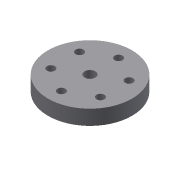
# Autodesk Inventor part: Window Motor Adapter
Saved by Autodesk Inventor 2015 (Build 190159000, 159)
## iProperties
Created: 2016-03-31
Part Number: Window Motor Adapter
Material: Generic
Document SubType Name: Modeling
Designer: Peter
Density: 1 g/cm^3
Appearance: Default
Author: Peter
Autodesk Inventor part; units mm, degrees
ref_plane "YZ Plane" through (0, 0, 0) normal (1, 0, 0) x (0, 1, 0)
sketch "Sketch1" plane through (0, 0, 0) normal (0, 0, 1) x (1, 0, 0)
  circle A0 centre (0, 0) radius 18.33
  arc A1 (-1.8, 7.7127) -> (-3.5788, 7.0653) centre (0, 0) ccw
  arc A2 (3.5788, 7.0653) -> (1.8, 7.7127) centre (0, 0) ccw
  arc A3 (7.3109, 3.0458) -> (6.3365, 4.7513) centre (0, 0) ccw
  arc A4 (7.5794, -2.2975) -> (7.9081, -0.4334) centre (0, 0) ccw
  arc A5 (4.3294, -6.632) -> (5.7794, -5.4152) centre (0, 0) ccw
  arc A6 (-0.9465, -7.8632) -> (0.9465, -7.8632) centre (0, 0) ccw
  arc A7 (-5.7794, -5.4152) -> (-4.3294, -6.632) centre (0, 0) ccw
  arc A8 (-6.3365, 4.7513) -> (-7.283, 3.112) centre (0, 0) ccw
  arc A9 (-7.9081, -0.4334) -> (-7.5794, -2.2975) centre (0, 0) ccw
  line L0 (-0.9465, -7.8632) -> (-2.2366, -11.4078)
  line L1 (-4.3294, -6.632) -> (-5.6195, -10.1765)
  line L2 (-5.6195, -10.1765) -> (-4.5495, -12.0298)
  line L3 (-2.2366, -11.4078) -> (-4.2475, -12.1397)
  arc A10 (-4.5495, -12.0298) -> (-4.2475, -12.1397) centre (-4.333, -11.9048) ccw
  line L4 (4.3294, -6.632) -> (5.6195, -10.1765)
  line L5 (0.9465, -7.8632) -> (2.2366, -11.4078)
  line L6 (2.2366, -11.4078) -> (4.2475, -12.1397)
  line L7 (5.6195, -10.1765) -> (4.5495, -12.0298)
  arc A11 (4.2475, -12.1397) -> (4.5495, -12.0298) centre (4.333, -11.9048) ccw
  line L8 (7.5794, -2.2975) -> (10.8461, -4.1836)
  line L9 (5.7794, -5.4152) -> (9.0461, -7.3012)
  line L10 (9.0461, -7.3012) -> (11.057, -6.5693)
  line L11 (10.8461, -4.1836) -> (11.2177, -6.291)
  arc A12 (11.057, -6.5693) -> (11.2177, -6.291) centre (10.9715, -6.3344) ccw
  line L12 (7.283, 3.112) -> (10.9978, 3.767)
  line L13 (7.9081, -0.4334) -> (11.6229, 0.2217)
  line L14 (11.6229, 0.2217) -> (12.6929, 2.0749)
  line L15 (10.9978, 3.767) -> (12.6371, 2.3914)
  arc A13 (12.6929, 2.0749) -> (12.6371, 2.3914) centre (12.4764, 2.1999) ccw
  line L16 (3.5788, 7.0653) -> (6.0034, 9.9549)
  line L17 (6.3365, 4.7513) -> (8.7612, 7.6408)
  line L18 (8.7612, 7.6408) -> (8.3896, 9.7483)
  line L19 (6.0034, 9.9549) -> (8.1434, 9.9549)
  arc A14 (8.3896, 9.7483) -> (8.1434, 9.9549) centre (8.1434, 9.7049) ccw
  line L20 (-1.8, 7.7127) -> (-1.8, 11.4848)
  line L21 (1.8, 7.7127) -> (1.8, 11.4848)
  line L22 (1.8, 11.4848) -> (0.1607, 12.8603)
  line L23 (-1.8, 11.4848) -> (-0.1607, 12.8603)
  arc A15 (0.1607, 12.8603) -> (-0.1607, 12.8603) centre (0, 12.6688) ccw
  line L24 (-6.3365, 4.7513) -> (-8.7612, 7.6408)
  line L25 (-3.5788, 7.0653) -> (-6.0034, 9.9549)
  line L26 (-6.0034, 9.9549) -> (-8.1434, 9.9549)
  line L27 (-8.7612, 7.6408) -> (-8.3896, 9.7483)
  arc A16 (-8.1434, 9.9549) -> (-8.3896, 9.7483) centre (-8.1434, 9.7049) ccw
  line L28 (-7.9081, -0.4334) -> (-11.6229, 0.2217)
  line L29 (-7.283, 3.112) -> (-10.9978, 3.767)
  line L30 (-10.9978, 3.767) -> (-12.6371, 2.3914)
  line L31 (-11.6229, 0.2217) -> (-12.6929, 2.0749)
  arc A17 (-12.6371, 2.3914) -> (-12.6929, 2.0749) centre (-12.4764, 2.1999) ccw
  line L32 (-5.7794, -5.4152) -> (-9.0461, -7.3012)
  line L33 (-7.5794, -2.2975) -> (-10.8461, -4.1836)
  line L34 (-10.8461, -4.1836) -> (-11.2177, -6.291)
  line L35 (-9.0461, -7.3012) -> (-11.057, -6.5693)
  arc A18 (-11.2177, -6.291) -> (-11.057, -6.5693) centre (-10.9715, -6.3344) ccw
  arc A19 (-0.9465, -7.8632) -> (0.9465, -7.8632) centre (0, 0) ccw
  arc A20 (4.3294, -6.632) -> (5.7794, -5.4152) centre (0, 0) ccw
  arc A21 (7.5794, -2.2975) -> (7.9081, -0.4334) centre (0, 0) ccw
  arc A22 (7.283, 3.112) -> (6.3365, 4.7513) centre (0, 0) ccw
  arc A23 (3.5788, 7.0653) -> (1.8, 7.7127) centre (0, 0) ccw
  arc A24 (-1.8, 7.7127) -> (-3.5788, 7.0653) centre (0, 0) ccw
  arc A25 (-6.3365, 4.7513) -> (-7.283, 3.112) centre (0, 0) ccw
  arc A26 (-7.9081, -0.4334) -> (-7.5794, -2.2975) centre (0, 0) ccw
  arc A27 (-5.7794, -5.4152) -> (-4.3294, -6.632) centre (0, 0) ccw
  point P0 (-2.306, -11.394)
  point P1 (-5.5574, -10.2106)
  dimension "d58" = 0.25
  dimension "d61" = 360
  constraints: 72 end point, 54 point on circle, 28 centre point, 2 coincident, 2 tangent, 109 other
  measures "d58" radius of A10
ref_plane "Work Plane1" through (0, 0, 10) normal (0, 0, 1) x (1, 0, 0)
sketch "Sketch2" plane through (0, 0, 10) normal (0, 0, 1) x (1, 0, 0)
  circle A0 centre (0, 0) radius 34.925
  circle A1 centre (0, 23.8125) radius 3.302
  circle A2 centre (-20.6222, 11.9063) radius 3.302
  circle A3 centre (-20.6222, -11.9062) radius 3.302
  circle A4 centre (0, -23.8125) radius 3.302
  circle A5 centre (20.6222, -11.9063) radius 3.302
  circle A6 centre (20.6222, 11.9062) radius 3.302
  dimension "d42" = 69.85
  dimension "d44" = 6.604
  dimension "d47" = 360
  constraints: 7 centre point, 1 coincident, 13 other
  measures "d42" diameter of A0
  measures "d44" diameter of A1
extrude "Extrusion2" add sketch "Sketch2" along normal blind 6.35
ref_plane "Work Plane2" through (0, 0, 10) normal (0, 0, -1) x (-1, 0, 0)
extrude "Extrusion4" add sketch "Sketch1" along normal up to surface (10 mm away)
sketch "Sketch4" plane through (0, 0, 10) normal (0, 0, -1) x (-1, 0, 0)
  circle A0 centre (0, 0) radius 4.5
  dimension "d65" = 9
  constraints: 1 centre point, 1 coincident
  measures "d65" diameter of A0
extrude "Extrusion5" cut sketch "Sketch4" against normal blind 10
fillet "Fillet1" radius 2 1 edges at (-18.33, 0, 10)
sketch "Sketch6" plane through (0, 0, 16.35) normal (0, 0, 1) x (1, 0, 0)
  circle A0 centre (0, 0) radius 34.925
  circle A1 centre (0, -23.8125) radius 3.302 projected
  circle A2 centre (0, -23.8125) radius 3.302
  circle A3 centre (20.6222, -11.9063) radius 3.302
  circle A4 centre (20.6222, 11.9062) radius 3.302
  circle A5 centre (0, 23.8125) radius 3.302
  circle A6 centre (-20.6222, 11.9063) radius 3.302
  circle A7 centre (-20.6222, -11.9062) radius 3.302
  dimension "d77" = 360
  constraints: 7 centre point, 2 coincident, 13 other
extrude "Extrusion7" add sketch "Sketch6" along normal blind 6.05
sketch "Sketch7" plane through (0, 0, 16.35) normal (0, 0, -1) x (-1, 0, 0)
  circle A0 centre (0, 0) radius 4.5
  constraints: 1 centre point, 1 coincident
extrude "Extrusion8" cut sketch "Sketch7" against normal up to surface (6.05 mm away)
chamfer "Chamfer1" distance 2 angle 45 1 edges at (4.5, 0, 10)
body "Solid1"
